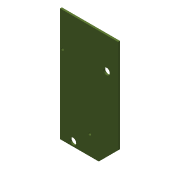
# Autodesk Inventor part: 01_PCBoard
Saved by Autodesk Inventor 2019 (Build 230136000, 136)
## iProperties
Created: 2016-11-08
Part Number: 01_PCBoard
Material: Generisch
Document SubType Name: Modeling
Designer: Bene
Density: 1 g/cm^3
Appearance: Olivgrün
Author: Bene
Autodesk Inventor part; units mm, degrees
ref_plane "YZ Plane" through (0, 0, 0) normal (1, 0, 0) x (0, 1, 0)
ref_plane "XZ Plane" through (0, 0, 0) normal (0, 1, 0) x (-1, 0, 0)
ref_plane "XY Plane" through (0, 0, 0) normal (0, 0, 1) x (1, 0, 0)
sketch "Skizze1" plane through (0, 0, 0) normal (0, 1, 0) x (-1, 0, 0)
  line L0 (0, 0) -> (-42, 0)
  line L1 (-63, 21) -> (-63, 123)
  line L2 (-63, 123) -> (0, 123)
  line L3 (0, 123) -> (0, 0)
  line L4 (-42, 0) -> (-63, 21)
  line L5 (-42, 0) -> (-12.3015, 0) construction
  circle A0 centre (-14, 5) radius 3.5
  circle A1 centre (-32, 21) radius 1.5
  circle A2 centre (-2.5, 86) radius 1.5
  circle A3 centre (-50.5, 89) radius 3.5
  dimension "d0" = 63
  dimension "d1" = 102
  dimension "d2" = 135
  dimension "d3" = 42
  dimension "d4" = 7
  dimension "d5" = 3
  dimension "d6" = 3
  dimension "d7" = 7
  dimension "d8" = 2.5
  dimension "d9" = 37
  dimension "d10" = 14
  dimension "d11" = 5
  dimension "d12" = 21
  dimension "d13" = 32
  dimension "d14" = 12.5
  dimension "d15" = 34
  constraints: 12 end point, 4 centre point, 2 horizontal, 2 parallel, 1 equal length, 1 perpendicular
  measures "d0" distance of L1.end L2.end
  measures "d1" distance of L1.start L1.end
  measures "d2" angle of L5 L4
  measures "d3" distance of L0.end L0.start
  measures "d4" diameter of A0
  measures "d5" diameter of A1
  measures "d6" diameter of A2
  measures "d7" diameter of A3
  measures "d8" distance from line of A2.centre L3
  measures "d9" distance from line of A2.centre L2
  measures "d10" distance from line of A0.centre L3
  measures "d11" distance from line of A0.centre L0
  measures "d12" distance from line of A1.centre L0
  measures "d13" distance from line of A1.centre L3
  measures "d14" distance from line of A3.centre L1
  measures "d15" distance from line of A3.centre L2
extrude "Extrusion1" add sketch "Skizze1" along normal blind 1
sketch "Sketch2" plane through (0, 1, 0) normal (0, 1, 0) x (1, 0, 0)
  circle A0 centre (50.5, -89) radius 3.5 projected
  circle A1 centre (14, -5) radius 3.5 projected
  circle A2 centre (2.5, -86) radius 1.5 projected
  circle A3 centre (32, -21) radius 1.5 projected
  line L0 (42, 0) -> (0, 0) projected
  line L1 (0, 0) -> (0, -123) projected
  line L2 (0, -123) -> (63, -123) projected
  line L3 (63, -123) -> (63, -21) projected
  line L4 (63, -21) -> (42, 0) projected
extrude "Extrusion2" add sketch "Sketch2" along normal blind 1
